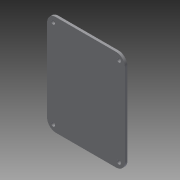
# Autodesk Inventor part: obudowa - budzik v4 dol dol
Saved by Autodesk Inventor 2014 (Build 180170000, 170)
## iProperties
Created: 2018-03-25
Part Number: obudowa - budzik v4 dol dol
Material: Generic
Document SubType Name: Modeling
Designer: HP820
Density: 1 g/cm^3
Appearance: Default
Author: HP820
Autodesk Inventor part; units mm, degrees
ref_plane "YZ Plane" through (0, 0, 0) normal (1, 0, 0) x (0, 1, 0)
ref_plane "XZ Plane" through (0, 0, 0) normal (0, 1, 0) x (-1, 0, 0)
ref_plane "XY Plane" through (0, 0, 0) normal (0, 0, 1) x (1, 0, 0)
sketch "Sketch1" plane through (0, 0, 0) normal (0, 1, 0) x (-1, 0, 0)
  circle A0 centre (29.5808, -39.6651) radius 1.75
  circle A1 centre (-29.5808, 39.6651) radius 1.75
  circle A2 centre (29.5808, 39.6651) radius 1.75
  circle A3 centre (-29.5808, -39.6651) radius 1.75
  line L0 (-27, -45) -> (27, -45)
  arc A4 (27, -45) -> (35, -37) centre (27, -37) ccw
  line L1 (35, -37) -> (35, 36.8048)
  ellipse E0 centre (27, 36.8048) end of major axis (27, 45) minor radius 8 (35, 36.8048) -> (27, 45) ccw
  line L2 (27, 45) -> (-27, 45)
  ellipse E1 centre (-27, 36.8048) end of major axis (-27, 45) minor radius 8 (-27, 45) -> (-35, 36.8048) ccw
  line L3 (-35, 36.8048) -> (-35, -37)
  arc A5 (-35, -37) -> (-27, -45) centre (-27, -37) ccw
  line L4 (22.5, -42.5) -> (-22.5, -42.5)
  arc A6 (-24.2843, -42.3395) -> (-22.5, -42.5) centre (-22.5, -32.5) ccw
  arc A7 (-24.2843, -42.3395) -> (-32.4877, -32.9952) centre (-33.2764, -41.9606) ccw
  arc A8 (-32.5, -32.5) -> (-32.4877, -32.9952) centre (-22.5, -32.5) ccw
  line L5 (-32.5, -32.5) -> (-32.5, 32.2561)
  ellipse E2 centre (-22.5, 32.2561) end of major axis (-22.5, 42.5) minor radius 10 (-32.4132, 33.603) -> (-32.5, 32.2561) ccw
  arc A9 (-32.4132, 33.603) -> (-23.6584, 42.431) centre (-32.6569, 42.5997) ccw
  ellipse E3 centre (-22.5, 32.2561) end of major axis (-22.5, 42.5) minor radius 10 (-22.5, 42.5) -> (-23.6584, 42.431) ccw
  line L6 (-22.5, 42.5) -> (22.5, 42.5)
  ellipse E4 centre (22.5, 32.2561) end of major axis (22.5, 42.5) minor radius 10 (23.6584, 42.431) -> (22.5, 42.5) ccw
  arc A10 (23.6584, 42.431) -> (32.4132, 33.603) centre (32.6569, 42.5997) ccw
  ellipse E5 centre (22.5, 32.2561) end of major axis (22.5, 42.5) minor radius 10 (32.5, 32.2561) -> (32.4132, 33.603) ccw
  line L7 (32.5, 32.2561) -> (32.5, -32.5)
  arc A11 (32.4877, -32.9952) -> (32.5, -32.5) centre (22.5, -32.5) ccw
  arc A12 (32.4877, -32.9952) -> (24.2843, -42.3395) centre (33.2764, -41.9606) ccw
  arc A13 (22.5, -42.5) -> (24.2843, -42.3395) centre (22.5, -32.5) ccw
  line L8 (-19.7694, -45) -> (13.1764, -45)
  point P0 (0, 0)
  point P1 (0, 0)
  constraints: 2 end point, 1 collinear, 6 other
extrude "Extrusion1" add sketch "Sketch1" along normal blind 2.2 contours A5 L3 E1 L2 E0 L1 A4 L0 | L4 A6 A7 A8 L5 E2 A9 E3 L6 E4 A10 E5 L7 A11 A12 A13
sketch "Sketch2" plane through (0, 2.2, 0) normal (0, 1, 0) x (1, 0, 0)
  line L0 (27, 45) -> (-27, 45) projected
  circle A0 centre (-25, 27) radius 1.25
  circle A1 centre (-25, 27) radius 3
  circle A2 centre (25, 27) radius 3
  circle A3 centre (25, 27) radius 1.25
  circle A4 centre (25, -33) radius 3
  circle A5 centre (25, -33) radius 1.25
  circle A6 centre (-25, -33) radius 3
  circle A7 centre (-25, -33) radius 1.25
  line L1 (-27, -45) -> (27, -45) projected
  point P0 (0, 0)
  point P1 (0, 0)
  point P2 (0, -5)
  dimension "d5" = 2.5
  dimension "d6" = 6
  dimension "d7" = 2.5
  dimension "d8" = 6
  dimension "d9" = 2.5
  dimension "d10" = 6
  dimension "d11" = 2.5
  dimension "d12" = 6
  dimension "d21" = 12
  dimension "d22" = 12
  dimension "d23" = 18
  dimension "d24" = 18
  constraints: 8 centre point, 4 coincident
  measures "d5" diameter of A0
  measures "d6" diameter of A1
  measures "d7" diameter of A3
  measures "d8" diameter of A2
  measures "d9" diameter of A5
  measures "d10" diameter of A4
  measures "d11" diameter of A7
  measures "d12" diameter of A6
  measures "d21" distance from line of L1 A4.centre
  measures "d22" distance from line of L1 A6.centre
  measures "d23" distance from line of A2.centre L0
  measures "d24" distance from line of L0 A0.centre
extrude "Extrusion2" add sketch "Sketch2" along normal blind 5
chamfer "Chamfer1" distance 2 angle 45 4 edges at (-28, 2.2, 33) (22, 2.2, 33) (-28, 2.2, -27) (22, 2.2, -27)
body "Solid1"
